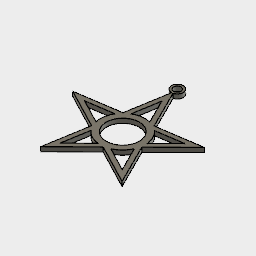
FPROJ_10 (Autodesk Fusion 360 design; units mm, degrees)
Autodesk Fusion 360 part; units mm, degrees
sketch "草图1" plane through (0, 0, 0) normal (0, 1, 0) x (1, 0, 0)
  line L0 (-18.7279, -36.0337) -> (2.3028, -15.3397)
  line L1 (2.3028, -15.3397) -> (28.4829, -28.9463)
  line L2 (28.4829, -28.9463) -> (15.3006, -2.5501)
  line L3 (15.3006, -2.5501) -> (36.3313, 18.1439)
  line L4 (7.1534, 13.7637) -> (36.3313, 18.1439)
  line L5 (7.1534, 13.7637) -> (-6.0289, 40.1599)
  line L6 (-6.0289, 40.1599) -> (-10.8795, 11.0565)
  line L7 (-40.0574, 6.6762) -> (-10.8795, 11.0565)
  line L8 (-40.0574, 6.6762) -> (-13.8773, -6.9304)
  line L9 (-13.8773, -6.9304) -> (-18.7279, -36.0337)
  line L10 (-30.4812, 5.0802) -> (-12.8573, 7.726)
  line L11 (10.0219, 11.1607) -> (27.6459, 13.8065)
  line L12 (-4.5877, 30.5593) -> (-7.5175, 12.9803)
  line L13 (-11.321, -9.8405) -> (-14.2508, -27.4195)
  line L14 (-30.4812, 5.0802) -> (-14.668, -3.1384)
  line L15 (5.8605, -13.8078) -> (21.6738, -22.0264)
  line L16 (-14.2508, -27.4195) -> (-1.5478, -14.9199)
  line L17 (14.943, 1.3069) -> (27.6459, 13.8065)
  line L18 (21.6738, -22.0264) -> (13.7114, -6.0826)
  line L19 (3.3747, 14.6154) -> (-4.5877, 30.5593)
  circle A0 centre (0, 0) radius 11
  arc A1 (-12.8573, 7.726) -> (-14.668, -3.1384) centre (0, 0) ccw
  arc A2 (3.3747, 14.6154) -> (-7.5175, 12.9803) centre (0, 0) ccw
  arc A3 (14.943, 1.3069) -> (10.0219, 11.1607) centre (0, 0) ccw
  arc A4 (-11.321, -9.8405) -> (-1.5478, -14.9199) centre (0, 0) ccw
  arc A5 (5.8605, -13.8078) -> (13.7114, -6.0826) centre (0, 0) ccw
  dimension "d3" = 30
  dimension "d8" = 22
  measures "d3" diameter of A4
  measures "d8" diameter of A0
sketch "草图3" plane through (0, 0, 0) normal (0, 1, 0) x (1, 0, 0)
  circle A0 centre (-75, 0) radius 2.5
  circle A1 centre (-75, 0) radius 4
  dimension "d4" = 5
  dimension "d5" = 8
  measures "d4" diameter of A0
  measures "d5" diameter of A1
extrude "拉伸1" add sketch "草图3" along normal blind 3 makes body 1
extrude "拉伸2" add sketch "草图1" along normal blind 3 separate body makes body 2
move_body "移动1" bodies 1 to x (1, 0, 0) y (0, 1, 0) z (0, 0, 1) at (69.0763, 0, -40.5763)
move_body "移动2" bodies 1 to x (1, 0, 0) y (0, 1, 0) z (0, 0, 1) at (-0.4652, 0, -2.1709)
combine "合并1" operation add target body 2 tool bodies 1
